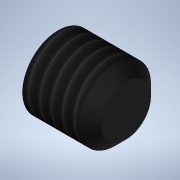
# Autodesk Inventor part: DIN-913 - M5x5
Saved by Autodesk Inventor 2021 (Build 250183000, 183)
## iProperties
Created: 2025-06-06
Part Number: DIN-913 - M5x5
Material: Generic
Catalog Web Link: www.cadenas.de
Description: DIN-913-Gewindestift
Vendor: FESTO
Document SubType Name: Modeling
Designer: psAdmin
Manufacturer: FESTO
Mass: 0.0823039 g
Surface Area: 1.23664 cm^2
Volume: 0.0823039 cm^3
Density: 1 g/cm^3
Appearance: PSOLRGB-175-175-175
Category: PARTsolutions
Company: FESTO
Title: DIN-913 - M5x5
Author: Cadenas PARTsolutions
Comments: Gewindestift
PSOL_IDENT_0: {$CADENAS_DATA/23d-libs/festo/zyl_zubeh/din_913/din_913.prj},171 {VTYP=3D},{NB=DIN-913 - M5x5},{LINA=
PSOL_IDENT_1: DIN-913 - M5x5},{NN=DIN-913},{DATE=22.07.2016 11:33:17},{GEOMDATE=22.07.2016 11:33:13},{VERSION=},{L
PSOL_IDENT_2: INEID=1040},{WBVAR=},{WBNUMERIC=}  {NB=DIN-913 - M5x5},{LINA=DIN-913 - M5x5},{KT=X},{IDNR=},{NENN=M5
PSOL_IDENT_3: x5},{D=5.000},{D3=4.019},{P=0.800},{L=5.000},{DP=3.500},{S=2.500},{T=2.000}
NB: DIN-913 - M5x5
NN: DIN-913
NT: Gewindestift
NBSYN: DIN-913 - $NENN.
LINA: DIN-913 - M5x5
CATALOG: Festo
ROWDESC: M5x5
D: 5
D3: 4.019
P: 0.8
L: 5
DP: 3.5
S: 2.5
T: 2
SUPPLIER: FESTO
ARTICLENO: DIN-913 - M5x5
BOMINFO: DIN-913 - M5x5
CREATOR: CADENAS GmbH
Autodesk Inventor part; units mm, degrees
sketch "Sketch_1" plane through (0, 0, 0) normal (0, 0, 1) x (1, 0, 0)
  line L0 (0.8333, 0) -> (5, 0)
  line L1 (5, 0) -> (5, -1.75)
  line L2 (5, -1.75) -> (4.25, -2.5)
  line L3 (4.25, -2.5) -> (0.2832, -2.5)
  line L4 (0.2832, -2.5) -> (0, -2.0095)
  line L5 (0, -2.0095) -> (0, -1.4434)
  line L6 (0, -1.4434) -> (0.8333, 0)
  line L7 (0.8333, 0) -> (5, 0)
  constraints: 16 end point
revolve "Revolution1" add sketch "Sketch_1" angle 360 about axis through (0.8333, 0, 0) along (1, 0, 0)
thread "Thread1" size "M5x0.8" class "6g" standard "ISO Metric profile" full length
sketch "Sketch_2" plane through (0, 0, 0) normal (1, 0, 0) x (0, 1, 0)
  line L0 (0, 1.4434) -> (-1.25, 0.7217)
  line L1 (-1.25, 0.7217) -> (-1.25, -0.7217)
  line L2 (-1.25, -0.7217) -> (0, -1.4434)
  line L3 (0, -1.4434) -> (1.25, -0.7217)
  line L4 (1.25, -0.7217) -> (1.25, 0.7217)
  line L5 (1.25, 0.7217) -> (0, 1.4434)
  constraints: 12 end point
extrude "Extrusion1" cut sketch "Sketch_2" along normal blind 2
ref_plane "IP1_XY" through (0, 0, 0) normal (1, 0, 0) x (0, 0, -1)
ref_plane "IP1_YZ" through (0, 0, 0) normal (0, 0, -1) x (0, 1, 0)
ref_plane "IP1_ZX" through (0, 0, 0) normal (0, 1, 0) x (1, 0, 0)
ref_plane "IP2_XY" through (5, 0, 0) normal (1, 0, 0) x (0, 0, -1)
ref_plane "IP2_YZ" through (5, 0, 0) normal (0, 0, -1) x (0, 1, 0)
ref_plane "IP2_ZX" through (5, 0, 0) normal (0, 1, 0) x (1, 0, 0)
body "Solid1"
